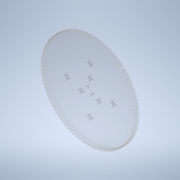
# Autodesk Inventor part: BigGear
Saved by Autodesk Inventor 2021 (Build 250183000, 183)
## iProperties
Created: 2022-02-16
Part Number: BigGear
Material: PMMA Plastic
Document SubType Name: Modeling
Designer: alexw
Mass: 170.04 g
Surface Area: 400.553 cm^2
Volume: 143.131 cm^3
Density: 1.188 g/cm^3
Appearance: Polycarbonate - Clear
BigGear_Flansch: 35,000 mm
Gear_Thick: 10,000 mm
GearDia: 162,338 mm
Dp_De_Diff_5: 1,140 mm
Author: alexw
Autodesk Inventor part; units mm, degrees
(part 1 of 2)
ref_plane "YZ Plane" through (0, 0, 0) normal (1, 0, 0) x (0, 1, 0)
ref_plane "XZ Plane" through (0, 0, 0) normal (0, 1, 0) x (-1, 0, 0)
sketch "Sketch1" plane through (0, 0, 0) normal (0, 0, 1) x (1, 0, 0)
  circle A0 centre (0, 0) radius 80.599
  circle A1 centre (0, 0) radius 6.925
  circle A2 centre (0, 0) radius 81.169 construction
  dimension "B_Gear_De" = 161.198
  dimension "d1" = 13.85
  dimension "BigGear_D" = 162.338
  constraints: 3 centre point, 3 coincident
  measures "B_Gear_De" diameter of A0
  measures "d1" diameter of A1
  measures "BigGear_D" diameter of A2
extrude "Extrusion1" add sketch "Sketch1" along normal blind 10
sketch "Sketch2" plane through (0, 0, 10) normal (0, 0, 1) x (1, 0, 0)
  line L0 (0, 17.5) -> (0, 0) construction
  circle A0 centre (0, 0) radius 17.5 construction
  point P0 (-15.1554, -8.75)
  point P1 (15.1554, -8.75)
  dimension "BigGear_Flansch" = 35
  dimension "d7" = 360
  constraints: 2 end point, 1 coincident, 1 vertical, 1 vertical alignment, 6 other
hole "Hole1" at (0, 17.5, 10) at (-15.1554, -8.75, 10) at (15.1554, -8.75, 10) direction (0, 0, -1) diameter 6.85 depth 11.8 tip angle 118
ref_plane "Work Plane1" through (0, 0, 5) normal (0, 0, 1) x (1, 0, 0)
sketch "Sketch3" plane through (0, 0, 10) normal (0, 0, 1) x (1, 0, 0)
  circle A0 centre (0, 0) radius 6.925 construction
  circle A1 centre (0, 0) radius 80.599 projected
  line L0 (0, 0) -> (0, 80.599) construction
  circle A2 centre (0, 0) radius 80.599 construction
  arc A3 (0.5699, 80.5902) -> (-0.5699, 80.5902) centre (0, 80.599) ccw construction
  arc A4 (0.5753, 80.4134) -> (2.4397, 78.6313) centre (2.4996, 80.5603) ccw
  arc A5 (-2.4397, 78.6313) -> (-0.5753, 80.4134) centre (-2.4996, 80.5603) ccw
  arc A6 (2.4996, 80.5603) -> (-2.4996, 80.5603) centre (0, 0) ccw construction
  line L1 (-2.4996, 80.5603) -> (-2.4397, 78.6313) construction
  line L2 (2.4996, 80.5603) -> (2.4397, 78.6313) construction
  line L3 (0, 80.599) -> (0, 81.169) construction
  arc A7 (2.4397, 78.6313) -> (-2.4397, 78.6313) centre (0, 0) ccw construction
  circle A8 centre (0, 0) radius 81.169 construction
  arc A9 (0.3768, 80.5981) -> (-0.3768, 80.5981) centre (0, 0) ccw
  arc A10 (-0.3768, 80.5981) -> (-0.5753, 80.4134) centre (-0.3759, 80.3981) ccw
  arc A11 (0.5753, 80.4134) -> (0.3768, 80.5981) centre (0.3759, 80.3981) ccw
  arc A12 (2.4055, 78.6323) -> (4.3761, 80.2963) centre (2.4645, 80.5613) ccw
  arc A13 (5.3378, 80.4221) -> (4.5856, 80.4685) centre (0, 0) ccw
  arc A14 (5.5245, 80.2254) -> (5.3378, 80.4221) centre (5.3245, 80.2225) ccw
  arc A15 (5.5245, 80.2254) -> (7.2757, 78.3319) centre (7.4542, 80.2536) ccw
  arc A16 (4.5856, 80.4685) -> (4.3761, 80.2963) centre (4.5742, 80.2688) ccw
  arc A17 (7.2416, 78.3351) -> (9.3109, 79.8746) centre (7.4193, 80.2568) ccw
  arc A18 (10.2785, 79.9409) -> (9.5306, 80.0336) centre (0, 0) ccw
  arc A19 (10.4528, 79.7332) -> (10.2785, 79.9409) centre (10.253, 79.7426) ccw
  arc A20 (10.4528, 79.7332) -> (12.0841, 77.7355) centre (12.3806, 79.6425) ccw
  arc A21 (9.5306, 80.0336) -> (9.3109, 79.8746) centre (9.507, 79.835) ccw
  arc A22 (12.0503, 77.7407) -> (14.2104, 79.1499) centre (12.3459, 79.6479) ccw
  arc A23 (15.1803, 79.1566) -> (14.4395, 79.295) centre (0, 0) ccw
  arc A24 (15.3414, 78.9385) -> (15.1803, 79.1566) centre (15.1426, 78.9601) ccw
  arc A25 (15.3414, 78.9385) -> (16.8467, 76.8441) centre (17.2599, 78.7293) ccw
  arc A26 (14.4395, 79.295) -> (14.2104, 79.1499) centre (14.4036, 79.0983) ccw
  arc A27 (16.8132, 76.8515) -> (19.056, 78.125) centre (17.2256, 78.7368) ccw
  arc A28 (20.0244, 78.0719) -> (19.2936, 78.2557) centre (0, 0) ccw
  arc A29 (20.1718, 77.8443) -> (20.0244, 78.0719) centre (19.9747, 77.8782) ccw
  arc A30 (20.1718, 77.8443) -> (21.5453, 75.6613) centre (22.0739, 77.5174) ccw
  arc A31 (19.2936, 78.2557) -> (19.056, 78.125) centre (19.2457, 78.0616) ccw
  arc A32 (21.5123, 75.6707) -> (23.8293, 76.8037) centre (22.0401, 77.527) ccw
  arc A33 (24.7926, 76.6911) -> (24.0745, 76.9196) centre (0, 0) ccw
  arc A34 (24.9258, 76.4549) -> (24.7926, 76.6911) centre (24.7311, 76.5008) ccw
  arc A35 (24.9258, 76.4549) -> (26.1622, 74.1914) centre (26.804, 76.0115) ccw
  arc A36 (24.0745, 76.9196) -> (23.8293, 76.8037) centre (24.0147, 76.7287) ccw
  arc A37 (26.1299, 74.2028) -> (28.5122, 75.1911) centre (26.7709, 76.0232) ccw
  arc A38 (29.4668, 75.0194) -> (28.764, 75.2916) centre (0, 0) ccw
  arc A39 (29.5851, 74.7754) -> (29.4668, 75.0194) centre (29.3937, 74.8333) ccw
  arc A40 (29.5851, 74.7754) -> (30.6799, 72.4401) centre (31.4325, 74.2172) ccw
  arc A41 (28.764, 75.2916) -> (28.5122, 75.1911) centre (28.6927, 75.1048) ccw
  arc A42 (30.6483, 72.4535) -> (33.087, 73.2932) centre (31.4002, 74.2309) ccw
  arc A43 (34.0291, 73.0631) -> (33.3445, 73.3781) centre (0, 0) ccw
  arc A44 (34.1322, 72.8123) -> (34.0291, 73.0631) centre (33.9447, 72.8818) ccw
  arc A45 (34.1322, 72.8123) -> (35.0812, 70.4141) centre (35.9418, 72.1415) ccw
  arc A46 (33.3445, 73.3781) -> (33.087, 73.2932) centre (33.2618, 73.196) ccw
  arc A47 (35.0505, 70.4293) -> (37.5362, 71.1173) centre (35.9104, 72.1571) ccw
  arc A48 (38.4624, 70.8297) -> (37.7985, 71.1862) centre (0, 0) ccw
  arc A49 (38.5499, 70.573) -> (38.4624, 70.8297) centre (38.367, 70.6539) ccw
  arc A50 (38.5499, 70.573) -> (39.3494, 68.1209) centre (40.3147, 69.792) ccw
  arc A51 (37.7985, 71.1862) -> (37.5362, 71.1173) centre (37.7047, 71.0096) ccw
  arc A52 (39.3197, 68.138) -> (41.8431, 68.6717) centre (40.2843, 69.8096) ccw
  arc A53 (42.7498, 68.3276) -> (42.1091, 68.7243) centre (0, 0) ccw
  arc A54 (42.8213, 68.066) -> (42.7498, 68.3276) centre (42.6437, 68.158) ccw
  arc A55 (42.8213, 68.066) -> (43.4684, 65.5693) centre (44.5347, 67.1778) ccw
  arc A56 (42.1091, 68.7243) -> (41.8431, 68.6717) centre (42.0046, 68.5538) ccw
  arc A57 (43.4398, 65.5882) -> (45.9912, 65.9655) centre (44.5054, 67.1972) ccw
  arc A58 (46.875, 65.5662) -> (46.2599, 66.0017) centre (0, 0) ccw
  arc A59 (46.9303, 65.3007) -> (46.875, 65.5662) centre (46.7587, 65.4035) ccw
  arc A60 (46.9303, 65.3007) -> (47.4224, 62.769) centre (48.5858, 64.3088) ccw
  arc A61 (46.2599, 66.0017) -> (45.9912, 65.9655) centre (46.1452, 65.8379) ccw
  arc A62 (47.3951, 62.7896) -> (49.9648, 63.0092) centre (48.5578, 64.33) ccw
  arc A63 (50.8225, 62.5562) -> (50.2353, 63.0287) centre (0, 0) ccw
  arc A64 (50.8613, 62.2878) -> (50.8225, 62.5562) centre (50.6963, 62.401) ccw
  arc A65 (50.8613, 62.2878) -> (51.1966, 59.7306) centre (52.4525, 61.1959) ccw
  arc A66 (50.2353, 63.0287) -> (49.9648, 63.0092) centre (50.1107, 62.8723) ccw
  arc A67 (51.1706, 59.7529) -> (53.749, 59.8138) centre (52.4259, 61.2187) ccw
  arc A68 (54.5771, 59.3089) -> (54.0201, 59.8166) centre (0, 0) ccw
  arc A69 (54.5993, 59.0386) -> (54.5771, 59.3089) centre (54.4417, 59.1617) ccw
  arc A70 (54.5993, 59.0386) -> (54.7765, 56.4656) centre (56.1203, 57.8508) ccw
  arc A71 (54.0201, 59.8166) -> (53.749, 59.8138) centre (53.8861, 59.6682) ccw
  arc A72 (54.7519, 56.4894) -> (57.3292, 56.3915) centre (56.0951, 57.8752) ccw
  arc A73 (58.1247, 55.8366) -> (57.6001, 56.3776) centre (0, 0) ccw
  arc A74 (58.1302, 55.5655) -> (58.1247, 55.8366) centre (57.9804, 55.698) ccw
  arc A75 (58.1302, 55.5655) -> (58.1487, 52.9864) centre (59.5752, 54.2862) ccw
  arc A76 (57.6001, 56.3776) -> (57.3292, 56.3915) centre (57.4571, 56.2377) ccw
  arc A77 (58.1256, 53.0117) -> (60.692, 52.7553) centre (59.5516, 54.3122) ccw
  arc A78 (61.4518, 52.1525) -> (60.9615, 52.7248) centre (0, 0) ccw
  arc A79 (61.4406, 51.8815) -> (61.4518, 52.1525) centre (61.2993, 52.0231) ccw
  arc A80 (61.4406, 51.8815) -> (61.3003, 49.3062) centre (62.8041, 50.5158) ccw
  arc A81 (60.9615, 52.7248) -> (60.692, 52.7553) centre (60.8102, 52.5939) ccw
  arc A82 (61.2788, 49.3329) -> (63.8246, 48.919) centre (62.7821, 50.5431) ccw
  arc A83 (64.5458, 48.2705) -> (64.0916, 48.8719) centre (0, 0) ccw
  arc A84 (64.5179, 48.0008) -> (64.5458, 48.2705) centre (64.3856, 48.1507) ccw
  arc A85 (64.5179, 48.0008) -> (64.2194, 45.439) centre (65.7948, 46.5537) ccw
  arc A86 (64.0916, 48.8719) -> (63.8246, 48.919) centre (63.9326, 48.7507) ccw
  arc A87 (64.1996, 45.4669) -> (66.715, 44.8971) centre (65.7745, 46.5823) ccw
  arc A88 (67.3949, 44.2055) -> (66.9787, 44.8337) centre (0, 0) ccw
  arc A89 (67.3505, 43.938) -> (67.3949, 44.2055) centre (67.2277, 44.0958) ccw
  arc A90 (67.3505, 43.938) -> (66.8949, 41.3994) centre (68.5359, 42.415) ccw
  arc A91 (66.9787, 44.8337) -> (66.715, 44.8971) centre (66.8125, 44.7225) ccw
  arc A92 (66.8768, 41.4285) -> (69.3524, 40.7049) centre (68.5174, 42.4448) ccw
  arc A93 (69.9884, 39.9727) -> (69.6116, 40.6254) centre (0, 0) ccw
  arc A94 (69.9277, 39.7085) -> (69.9884, 39.9727) centre (69.8148, 39.8736) ccw
  arc A95 (69.9277, 39.7085) -> (69.3166, 37.2028) centre (71.017, 38.1154) ccw
  arc A96 (69.6116, 40.6254) -> (69.3524, 40.7049) centre (69.4389, 40.5246) ccw
  arc A97 (69.3003, 37.233) -> (71.7267, 36.3583) centre (71.0004, 38.1463) ccw
  arc A98 (72.3165, 35.5884) -> (71.9805, 36.263) centre (0, 0) ccw
  arc A99 (72.2395, 35.3283) -> (72.3165, 35.5884) centre (72.137, 35.5001) ccw
  arc A100 (72.2395, 35.3283) -> (71.4753, 32.865) centre (73.2287, 33.6712) ccw
  arc A101 (71.9805, 36.263) -> (71.7267, 36.3583) centre (71.8019, 36.173) ccw
  arc A102 (71.461, 32.8961) -> (73.8289, 31.8738) centre (73.2141, 33.7031) ccw
  arc A103 (74.3701, 31.069) -> (74.0764, 31.763) centre (0, 0) ccw
  arc A104 (74.2774, 30.8142) -> (74.3701, 31.069) centre (74.1856, 30.9919) ccw
  arc A105 (74.2774, 30.8142) -> (73.363, 28.4026) centre (75.1627, 29.0994) ccw
  arc A106 (74.0764, 31.763) -> (73.8289, 31.8738) centre (73.8926, 31.6842) ccw
  arc A107 (73.3506, 28.4345) -> (75.651, 27.2684) centre (75.15, 29.1321) ccw
  arc A108 (76.1417, 26.4318) -> (75.8913, 27.1426) centre (0, 0) ccw
  arc A109 (76.0334, 26.1832) -> (76.1417, 26.4318) centre (75.9528, 26.3662) ccw
  arc A110 (76.0334, 26.1832) -> (74.9723, 23.8324) centre (76.8115, 24.4171) ccw
  arc A111 (75.8913, 27.1426) -> (75.651, 27.2684) centre (75.7029, 27.0752) ccw
  arc A112 (74.9619, 23.8651) -> (77.1862, 22.5595) centre (76.8009, 24.4505) ccw
  arc A113 (77.6245, 21.6943) -> (77.4182, 22.4192) centre (0, 0) ccw
  arc A114 (77.5011, 21.4528) -> (77.6245, 21.6943) centre (77.4319, 21.6405) ccw
  arc A115 (77.5011, 21.4528) -> (76.2973, 19.1719) centre (78.169, 19.6422) ccw
  arc A116 (77.4182, 22.4192) -> (77.1862, 22.5595) centre (77.2261, 22.3635) ccw
  arc A117 (76.2889, 19.2051) -> (78.4286, 17.7651) centre (78.1604, 19.6762) ccw
  arc A118 (78.8128, 16.8745) -> (78.6515, 17.6107) centre (0, 0) ccw
  arc A119 (78.6747, 16.6411) -> (78.8128, 16.8745) centre (78.6172, 16.8326) ccw
  arc A120 (78.6747, 16.6411) -> (77.3328, 14.4386) centre (79.2299, 14.7928) ccw
  arc A121 (78.6515, 17.6107) -> (78.4286, 17.7651) centre (78.4564, 17.567) ccw
  arc A122 (77.3265, 14.4723) -> (79.3735, 12.9032) centre (79.2234, 14.8273) ccw
  arc A123 (79.7021, 11.9907) -> (79.5865, 12.7354) centre (0, 0) ccw
  arc A124 (79.55, 11.7663) -> (79.7021, 11.9907) centre (79.5043, 11.961) ccw
  arc A125 (79.55, 11.7663) -> (78.075, 9.6505) centre (79.9903, 9.8873) ccw
  arc A126 (79.5865, 12.7354) -> (79.3735, 12.9032) centre (79.389, 12.7038) ccw
  arc A127 (78.0707, 9.6845) -> (80.0173, 7.9925) centre (79.986, 9.9221) ccw
  arc A128 (80.2891, 7.0615) -> (80.2196, 7.8119) centre (0, 0) ccw
  arc A129 (80.1234, 6.8468) -> (80.2891, 7.0615) centre (80.0899, 7.0439) ccw
  arc A130 (80.1234, 6.8468) -> (78.521, 4.8258) centre (80.4472, 4.9442) ccw
  arc A131 (80.2196, 7.8119) -> (80.0173, 7.9925) centre (80.0205, 7.7925) ccw
  arc A132 (78.5189, 4.86) -> (80.3575, 3.0514) centre (80.4451, 4.9793) ccw
  arc A133 (80.5715, 2.1054) -> (80.5483, 2.8587) centre (0, 0) ccw
  arc A134 (80.3929, 1.9013) -> (80.5715, 2.1054) centre (80.3716, 2.1002) ccw
  arc A135 (80.3929, 1.9013) -> (78.6691, -0.0171) centre (80.599, -0.0176) ccw
  arc A136 (80.5483, 2.8587) -> (80.3575, 3.0514) centre (80.3484, 2.8516) ccw
  arc A137 (78.6691, 0.0171) -> (80.3929, -1.9013) centre (80.599, 0.0176) ccw
  arc A138 (80.5483, -2.8587) -> (80.5715, -2.1054) centre (0, 0) ccw
  arc A139 (80.3575, -3.0514) -> (80.5483, -2.8587) centre (80.3484, -2.8516) ccw
  arc A140 (80.3575, -3.0514) -> (78.5189, -4.86) centre (80.4451, -4.9793) ccw
  arc A141 (80.5715, -2.1054) -> (80.3929, -1.9013) centre (80.3716, -2.1002) ccw
  arc A142 (78.521, -4.8258) -> (80.1234, -6.8468) centre (80.4472, -4.9442) ccw
  arc A143 (80.2196, -7.8119) -> (80.2891, -7.0615) centre (0, 0) ccw
  arc A144 (80.0173, -7.9925) -> (80.2196, -7.8119) centre (80.0205, -7.7925) ccw
  arc A145 (80.0173, -7.9925) -> (78.0707, -9.6845) centre (79.986, -9.9221) ccw
  arc A146 (80.2891, -7.0615) -> (80.1234, -6.8468) centre (80.0899, -7.0439) ccw
  arc A147 (78.075, -9.6505) -> (79.55, -11.7663) centre (79.9903, -9.8873) ccw
  arc A148 (79.5865, -12.7354) -> (79.7021, -11.9907) centre (0, 0) ccw
  arc A149 (79.3735, -12.9032) -> (79.5865, -12.7354) centre (79.389, -12.7038) ccw
  arc A150 (79.3735, -12.9032) -> (77.3265, -14.4723) centre (79.2234, -14.8273) ccw
  arc A151 (79.7021, -11.9907) -> (79.55, -11.7663) centre (79.5043, -11.961) ccw
  arc A152 (77.3328, -14.4386) -> (78.6747, -16.6411) centre (79.2299, -14.7928) ccw
  arc A153 (78.6515, -17.6107) -> (78.8128, -16.8745) centre (0, 0) ccw
  arc A154 (78.4286, -17.7651) -> (78.6515, -17.6107) centre (78.4564, -17.567) ccw
  arc A155 (78.4286, -17.7651) -> (76.2889, -19.2051) centre (78.1604, -19.6762) ccw
  arc A156 (78.8128, -16.8745) -> (78.6747, -16.6411) centre (78.6172, -16.8326) ccw
  arc A157 (76.2973, -19.1719) -> (77.5011, -21.4528) centre (78.169, -19.6422) ccw
  arc A158 (77.4182, -22.4192) -> (77.6245, -21.6943) centre (0, 0) ccw
  arc A159 (77.1862, -22.5595) -> (77.4182, -22.4192) centre (77.2261, -22.3635) ccw
  arc A160 (77.1862, -22.5595) -> (74.9619, -23.8651) centre (76.8009, -24.4505) ccw
  arc A161 (77.6245, -21.6943) -> (77.5011, -21.4528) centre (77.4319, -21.6405) ccw
  arc A162 (74.9723, -23.8324) -> (76.0334, -26.1832) centre (76.8115, -24.4171) ccw
  arc A163 (75.8913, -27.1426) -> (76.1417, -26.4318) centre (0, 0) ccw
  arc A164 (75.651, -27.2684) -> (75.8913, -27.1426) centre (75.7029, -27.0752) ccw
  arc A165 (75.651, -27.2684) -> (73.3506, -28.4345) centre (75.15, -29.1321) ccw
  arc A166 (76.1417, -26.4318) -> (76.0334, -26.1832) centre (75.9528, -26.3662) ccw
  arc A167 (73.363, -28.4026) -> (74.2774, -30.8142) centre (75.1627, -29.0994) ccw
  arc A168 (74.0764, -31.763) -> (74.3701, -31.069) centre (0, 0) ccw
  arc A169 (73.8289, -31.8738) -> (74.0764, -31.763) centre (73.8926, -31.6842) ccw
  arc A170 (73.8289, -31.8738) -> (71.461, -32.8961) centre (73.2141, -33.7031) ccw
  arc A171 (74.3701, -31.069) -> (74.2774, -30.8142) centre (74.1856, -30.9919) ccw
  arc A172 (71.4753, -32.865) -> (72.2395, -35.3283) centre (73.2287, -33.6712) ccw
  arc A173 (71.9805, -36.263) -> (72.3165, -35.5884) centre (0, 0) ccw
  arc A174 (71.7267, -36.3583) -> (71.9805, -36.263) centre (71.8019, -36.173) ccw
  arc A175 (71.7267, -36.3583) -> (69.3003, -37.233) centre (71.0004, -38.1463) ccw
  arc A176 (72.3165, -35.5884) -> (72.2395, -35.3283) centre (72.137, -35.5001) ccw
  arc A177 (69.3166, -37.2028) -> (69.9277, -39.7085) centre (71.017, -38.1154) ccw
  arc A178 (69.6116, -40.6254) -> (69.9884, -39.9727) centre (0, 0) ccw
  arc A179 (69.3524, -40.7049) -> (69.6116, -40.6254) centre (69.4389, -40.5246) ccw
  arc A180 (69.3524, -40.7049) -> (66.8768, -41.4285) centre (68.5174, -42.4448) ccw
  arc A181 (69.9884, -39.9727) -> (69.9277, -39.7085) centre (69.8148, -39.8736) ccw
  arc A182 (66.8949, -41.3994) -> (67.3505, -43.938) centre (68.5359, -42.415) ccw
  arc A183 (66.9787, -44.8337) -> (67.3949, -44.2055) centre (0, 0) ccw
  arc A184 (66.715, -44.8971) -> (66.9787, -44.8337) centre (66.8125, -44.7225) ccw
  arc A185 (66.715, -44.8971) -> (64.1996, -45.4669) centre (65.7745, -46.5823) ccw
  arc A186 (67.3949, -44.2055) -> (67.3505, -43.938) centre (67.2277, -44.0958) ccw
  arc A187 (64.2194, -45.439) -> (64.5179, -48.0008) centre (65.7948, -46.5537) ccw
  arc A188 (64.0916, -48.8719) -> (64.5458, -48.2705) centre (0, 0) ccw
  arc A189 (63.8246, -48.919) -> (64.0916, -48.8719) centre (63.9326, -48.7507) ccw
  arc A190 (63.8246, -48.919) -> (61.2788, -49.3329) centre (62.7821, -50.5431) ccw
  arc A191 (64.5458, -48.2705) -> (64.5179, -48.0008) centre (64.3856, -48.1507) ccw
  arc A192 (61.3003, -49.3062) -> (61.4406, -51.8815) centre (62.8041, -50.5158) ccw
  arc A193 (60.9615, -52.7248) -> (61.4518, -52.1525) centre (0, 0) ccw
  arc A194 (60.692, -52.7553) -> (60.9615, -52.7248) centre (60.8102, -52.5939) ccw
  arc A195 (60.692, -52.7553) -> (58.1256, -53.0117) centre (59.5516, -54.3122) ccw
  arc A196 (61.4518, -52.1525) -> (61.4406, -51.8815) centre (61.2993, -52.0231) ccw
  arc A197 (58.1487, -52.9864) -> (58.1302, -55.5655) centre (59.5752, -54.2862) ccw
  arc A198 (57.6001, -56.3776) -> (58.1247, -55.8366) centre (0, 0) ccw
  arc A199 (57.3292, -56.3915) -> (57.6001, -56.3776) centre (57.4571, -56.2377) ccw
  arc A200 (57.3292, -56.3915) -> (54.7519, -56.4894) centre (56.0951, -57.8752) ccw
  arc A201 (58.1247, -55.8366) -> (58.1302, -55.5655) centre (57.9804, -55.698) ccw
  arc A202 (54.7765, -56.4656) -> (54.5993, -59.0386) centre (56.1203, -57.8508) ccw
  arc A203 (54.0201, -59.8166) -> (54.5771, -59.3089) centre (0, 0) ccw
  arc A204 (53.749, -59.8138) -> (54.0201, -59.8166) centre (53.8861, -59.6682) ccw
  arc A205 (53.749, -59.8138) -> (51.1706, -59.7529) centre (52.4259, -61.2187) ccw
  arc A206 (54.5771, -59.3089) -> (54.5993, -59.0386) centre (54.4417, -59.1617) ccw
  arc A207 (51.1966, -59.7306) -> (50.8613, -62.2878) centre (52.4525, -61.1959) ccw
  arc A208 (50.2353, -63.0287) -> (50.8225, -62.5562) centre (0, 0) ccw
  arc A209 (49.9648, -63.0092) -> (50.2353, -63.0287) centre (50.1107, -62.8723) ccw
  arc A210 (49.9648, -63.0092) -> (47.3951, -62.7896) centre (48.5578, -64.33) ccw
  arc A211 (50.8225, -62.5562) -> (50.8613, -62.2878) centre (50.6963, -62.401) ccw
  arc A212 (47.4224, -62.769) -> (46.9303, -65.3007) centre (48.5858, -64.3088) ccw
  arc A213 (46.2599, -66.0017) -> (46.875, -65.5662) centre (0, 0) ccw
  arc A214 (45.9912, -65.9655) -> (46.2599, -66.0017) centre (46.1452, -65.8379) ccw
  arc A215 (45.9912, -65.9655) -> (43.4398, -65.5882) centre (44.5054, -67.1972) ccw
  arc A216 (46.875, -65.5662) -> (46.9303, -65.3007) centre (46.7587, -65.4035) ccw
  arc A217 (43.4684, -65.5693) -> (42.8213, -68.066) centre (44.5347, -67.1778) ccw
  arc A218 (42.1091, -68.7243) -> (42.7498, -68.3276) centre (0, 0) ccw
  arc A219 (41.8431, -68.6717) -> (42.1091, -68.7243) centre (42.0046, -68.5538) ccw
  arc A220 (41.8431, -68.6717) -> (39.3197, -68.138) centre (40.2843, -69.8096) ccw
  arc A221 (42.7498, -68.3276) -> (42.8213, -68.066) centre (42.6437, -68.158) ccw
  arc A222 (39.3494, -68.1209) -> (38.5499, -70.573) centre (40.3147, -69.792) ccw
  arc A223 (37.7985, -71.1862) -> (38.4624, -70.8297) centre (0, 0) ccw
  arc A224 (37.5362, -71.1173) -> (37.7985, -71.1862) centre (37.7047, -71.0096) ccw
  arc A225 (37.5362, -71.1173) -> (35.0505, -70.4293) centre (35.9104, -72.1571) ccw
  arc A226 (38.4624, -70.8297) -> (38.5499, -70.573) centre (38.367, -70.6539) ccw
  arc A227 (35.0812, -70.4141) -> (34.1322, -72.8123) centre (35.9418, -72.1415) ccw
  arc A228 (33.3445, -73.3781) -> (34.0291, -73.0631) centre (0, 0) ccw
  arc A229 (33.087, -73.2932) -> (33.3445, -73.3781) centre (33.2618, -73.196) ccw
  arc A230 (33.087, -73.2932) -> (30.6483, -72.4535) centre (31.4002, -74.2309) ccw
  arc A231 (34.0291, -73.0631) -> (34.1322, -72.8123) centre (33.9447, -72.8818) ccw
  arc A232 (30.6799, -72.4401) -> (29.5851, -74.7754) centre (31.4325, -74.2172) ccw
  arc A233 (28.764, -75.2916) -> (29.4668, -75.0194) centre (0, 0) ccw
  arc A234 (28.5122, -75.1911) -> (28.764, -75.2916) centre (28.6927, -75.1048) ccw
  arc A235 (28.5122, -75.1911) -> (26.1299, -74.2028) centre (26.7709, -76.0232) ccw
  arc A236 (29.4668, -75.0194) -> (29.5851, -74.7754) centre (29.3937, -74.8333) ccw
  arc A237 (26.1622, -74.1914) -> (24.9258, -76.4549) centre (26.804, -76.0115) ccw
  arc A238 (24.0745, -76.9196) -> (24.7926, -76.6911) centre (0, 0) ccw
  arc A239 (23.8293, -76.8037) -> (24.0745, -76.9196) centre (24.0147, -76.7287) ccw
  arc A240 (23.8293, -76.8037) -> (21.5123, -75.6707) centre (22.0401, -77.527) ccw
  arc A241 (24.7926, -76.6911) -> (24.9258, -76.4549) centre (24.7311, -76.5008) ccw
  arc A242 (21.5453, -75.6613) -> (20.1718, -77.8443) centre (22.0739, -77.5174) ccw
  arc A243 (19.2936, -78.2557) -> (20.0244, -78.0719) centre (0, 0) ccw
  arc A244 (19.056, -78.125) -> (19.2936, -78.2557) centre (19.2457, -78.0616) ccw
  arc A245 (19.056, -78.125) -> (16.8132, -76.8515) centre (17.2256, -78.7368) ccw
  arc A246 (20.0244, -78.0719) -> (20.1718, -77.8443) centre (19.9747, -77.8782) ccw
  arc A247 (16.8467, -76.8441) -> (15.3414, -78.9385) centre (17.2599, -78.7293) ccw
  arc A248 (14.4395, -79.295) -> (15.1803, -79.1566) centre (0, 0) ccw
  arc A249 (14.2104, -79.1499) -> (14.4395, -79.295) centre (14.4036, -79.0983) ccw
  arc A250 (14.2104, -79.1499) -> (12.0503, -77.7407) centre (12.3459, -79.6479) ccw
  arc A251 (15.1803, -79.1566) -> (15.3414, -78.9385) centre (15.1426, -78.9601) ccw
  arc A252 (12.0841, -77.7355) -> (10.4528, -79.7332) centre (12.3806, -79.6425) ccw
  arc A253 (9.5306, -80.0336) -> (10.2785, -79.9409) centre (0, 0) ccw
  arc A254 (9.3109, -79.8746) -> (9.5306, -80.0336) centre (9.507, -79.835) ccw
  arc A255 (9.3109, -79.8746) -> (7.2416, -78.3351) centre (7.4193, -80.2568) ccw
  arc A256 (10.2785, -79.9409) -> (10.4528, -79.7332) centre (10.253, -79.7426) ccw
  arc A257 (7.2757, -78.3319) -> (5.5245, -80.2254) centre (7.4542, -80.2536) ccw
  arc A258 (4.5856, -80.4685) -> (5.3378, -80.4221) centre (0, 0) ccw
  arc A259 (4.3761, -80.2963) -> (4.5856, -80.4685) centre (4.5742, -80.2688) ccw
  arc A260 (4.3761, -80.2963) -> (2.4055, -78.6323) centre (2.4645, -80.5613) ccw
  arc A261 (5.3378, -80.4221) -> (5.5245, -80.2254) centre (5.3245, -80.2225) ccw
  arc A262 (2.4397, -78.6313) -> (0.5753, -80.4134) centre (2.4996, -80.5603) ccw
  arc A263 (-0.3768, -80.5981) -> (0.3768, -80.5981) centre (0, 0) ccw
  arc A264 (-0.5753, -80.4134) -> (-0.3768, -80.5981) centre (-0.3759, -80.3981) ccw
  arc A265 (-0.5753, -80.4134) -> (-2.4397, -78.6313) centre (-2.4996, -80.5603) ccw
  arc A266 (0.3768, -80.5981) -> (0.5753, -80.4134) centre (0.3759, -80.3981) ccw
  arc A267 (-2.4055, -78.6323) -> (-4.3761, -80.2963) centre (-2.4645, -80.5613) ccw
  arc A268 (-5.3378, -80.4221) -> (-4.5856, -80.4685) centre (0, 0) ccw
  arc A269 (-5.5245, -80.2254) -> (-5.3378, -80.4221) centre (-5.3245, -80.2225) ccw
  arc A270 (-5.5245, -80.2254) -> (-7.2757, -78.3319) centre (-7.4542, -80.2536) ccw
  arc A271 (-4.5856, -80.4685) -> (-4.3761, -80.2963) centre (-4.5742, -80.2688) ccw
  arc A272 (-7.2416, -78.3351) -> (-9.3109, -79.8746) centre (-7.4193, -80.2568) ccw
  arc A273 (-10.2785, -79.9409) -> (-9.5306, -80.0336) centre (0, 0) ccw
  arc A274 (-10.4528, -79.7332) -> (-10.2785, -79.9409) centre (-10.253, -79.7426) ccw
  arc A275 (-10.4528, -79.7332) -> (-12.0841, -77.7355) centre (-12.3806, -79.6425) ccw
  arc A276 (-9.5306, -80.0336) -> (-9.3109, -79.8746) centre (-9.507, -79.835) ccw
  arc A277 (-12.0503, -77.7407) -> (-14.2104, -79.1499) centre (-12.3459, -79.6479) ccw
  arc A278 (-15.1803, -79.1566) -> (-14.4395, -79.295) centre (0, 0) ccw
  arc A279 (-15.3414, -78.9385) -> (-15.1803, -79.1566) centre (-15.1426, -78.9601) ccw
  arc A280 (-15.3414, -78.9385) -> (-16.8467, -76.8441) centre (-17.2599, -78.7293) ccw
  arc A281 (-14.4395, -79.295) -> (-14.2104, -79.1499) centre (-14.4036, -79.0983) ccw
  arc A282 (-16.8132, -76.8515) -> (-19.056, -78.125) centre (-17.2256, -78.7368) ccw
  arc A283 (-20.0244, -78.0719) -> (-19.2936, -78.2557) centre (0, 0) ccw
  arc A284 (-20.1718, -77.8443) -> (-20.0244, -78.0719) centre (-19.9747, -77.8782) ccw
  arc A285 (-20.1718, -77.8443) -> (-21.5453, -75.6613) centre (-22.0739, -77.5174) ccw
  arc A286 (-19.2936, -78.2557) -> (-19.056, -78.125) centre (-19.2457, -78.0616) ccw
  arc A287 (-21.5123, -75.6707) -> (-23.8293, -76.8037) centre (-22.0401, -77.527) ccw
  arc A288 (-24.7926, -76.6911) -> (-24.0745, -76.9196) centre (0, 0) ccw
  arc A289 (-24.9258, -76.4549) -> (-24.7926, -76.6911) centre (-24.7311, -76.5008) ccw
  arc A290 (-24.9258, -76.4549) -> (-26.1622, -74.1914) centre (-26.804, -76.0115) ccw
  arc A291 (-24.0745, -76.9196) -> (-23.8293, -76.8037) centre (-24.0147, -76.7287) ccw
  arc A292 (-26.1299, -74.2028) -> (-28.5122, -75.1911) centre (-26.7709, -76.0232) ccw
  arc A293 (-29.4668, -75.0194) -> (-28.764, -75.2916) centre (0, 0) ccw
  arc A294 (-29.5851, -74.7754) -> (-29.4668, -75.0194) centre (-29.3937, -74.8333) ccw
  arc A295 (-29.5851, -74.7754) -> (-30.6799, -72.4401) centre (-31.4325, -74.2172) ccw
  arc A296 (-28.764, -75.2916) -> (-28.5122, -75.1911) centre (-28.6927, -75.1048) ccw
  arc A297 (-30.6483, -72.4535) -> (-33.087, -73.2932) centre (-31.4002, -74.2309) ccw
  arc A298 (-34.0291, -73.0631) -> (-33.3445, -73.3781) centre (0, 0) ccw
  arc A299 (-34.1322, -72.8123) -> (-34.0291, -73.0631) centre (-33.9447, -72.8818) ccw
  arc A300 (-34.1322, -72.8123) -> (-35.0812, -70.4141) centre (-35.9418, -72.1415) ccw
  arc A301 (-33.3445, -73.3781) -> (-33.087, -73.2932) centre (-33.2618, -73.196) ccw
  arc A302 (-35.0505, -70.4293) -> (-37.5362, -71.1173) centre (-35.9104, -72.1571) ccw
  arc A303 (-38.4624, -70.8297) -> (-37.7985, -71.1862) centre (0, 0) ccw
  arc A304 (-38.5499, -70.573) -> (-38.4624, -70.8297) centre (-38.367, -70.6539) ccw
  arc A305 (-38.5499, -70.573) -> (-39.3494, -68.1209) centre (-40.3147, -69.792) ccw
  arc A306 (-37.7985, -71.1862) -> (-37.5362, -71.1173) centre (-37.7047, -71.0096) ccw
  arc A307 (-39.3197, -68.138) -> (-41.8431, -68.6717) centre (-40.2843, -69.8096) ccw
  arc A308 (-42.7498, -68.3276) -> (-42.1091, -68.7243) centre (0, 0) ccw
  arc A309 (-42.8213, -68.066) -> (-42.7498, -68.3276) centre (-42.6437, -68.158) ccw
  arc A310 (-42.8213, -68.066) -> (-43.4684, -65.5693) centre (-44.5347, -67.1778) ccw
  arc A311 (-42.1091, -68.7243) -> (-41.8431, -68.6717) centre (-42.0046, -68.5538) ccw
  arc A312 (-43.4398, -65.5882) -> (-45.9912, -65.9655) centre (-44.5054, -67.1972) ccw
  arc A313 (-46.875, -65.5662) -> (-46.2599, -66.0017) centre (0, 0) ccw
  arc A314 (-46.9303, -65.3007) -> (-46.875, -65.5662) centre (-46.7587, -65.4035) ccw
  arc A315 (-46.9303, -65.3007) -> (-47.4224, -62.769) centre (-48.5858, -64.3088) ccw
  arc A316 (-46.2599, -66.0017) -> (-45.9912, -65.9655) centre (-46.1452, -65.8379) ccw
  arc A317 (-47.3951, -62.7896) -> (-49.9648, -63.0092) centre (-48.5578, -64.33) ccw
  arc A318 (-50.8225, -62.5562) -> (-50.2353, -63.0287) centre (0, 0) ccw
  arc A319 (-50.8613, -62.2878) -> (-50.8225, -62.5562) centre (-50.6963, -62.401) ccw
  arc A320 (-50.8613, -62.2878) -> (-51.1966, -59.7306) centre (-52.4525, -61.1959) ccw
  arc A321 (-50.2353, -63.0287) -> (-49.9648, -63.0092) centre (-50.1107, -62.8723) ccw
  arc A322 (-51.1706, -59.7529) -> (-53.749, -59.8138) centre (-52.4259, -61.2187) ccw
  arc A323 (-54.5771, -59.3089) -> (-54.0201, -59.8166) centre (0, 0) ccw
  arc A324 (-54.5993, -59.0386) -> (-54.5771, -59.3089) centre (-54.4417, -59.1617) ccw
  arc A325 (-54.5993, -59.0386) -> (-54.7765, -56.4656) centre (-56.1203, -57.8508) ccw
  arc A326 (-54.0201, -59.8166) -> (-53.749, -59.8138) centre (-53.8861, -59.6682) ccw
  arc A327 (-54.7519, -56.4894) -> (-57.3292, -56.3915) centre (-56.0951, -57.8752) ccw
  arc A328 (-58.1247, -55.8366) -> (-57.6001, -56.3776) centre (0, 0) ccw
  arc A329 (-58.1302, -55.5655) -> (-58.1247, -55.8366) centre (-57.9804, -55.698) ccw
  arc A330 (-58.1302, -55.5655) -> (-58.1487, -52.9864) centre (-59.5752, -54.2862) ccw
  arc A331 (-57.6001, -56.3776) -> (-57.3292, -56.3915) centre (-57.4571, -56.2377) ccw
  arc A332 (-58.1256, -53.0117) -> (-60.692, -52.7553) centre (-59.5516, -54.3122) ccw
  arc A333 (-61.4518, -52.1525) -> (-60.9615, -52.7248) centre (0, 0) ccw
  arc A334 (-61.4406, -51.8815) -> (-61.4518, -52.1525) centre (-61.2993, -52.0231) ccw
  arc A335 (-61.4406, -51.8815) -> (-61.3003, -49.3062) centre (-62.8041, -50.5158) ccw
  arc A336 (-60.9615, -52.7248) -> (-60.692, -52.7553) centre (-60.8102, -52.5939) ccw
  arc A337 (-61.2788, -49.3329) -> (-63.8246, -48.919) centre (-62.7821, -50.5431) ccw
  arc A338 (-64.5458, -48.2705) -> (-64.0916, -48.8719) centre (0, 0) ccw
  arc A339 (-64.5179, -48.0008) -> (-64.5458, -48.2705) centre (-64.3856, -48.1507) ccw
  arc A340 (-64.5179, -48.0008) -> (-64.2194, -45.439) centre (-65.7948, -46.5537) ccw
  arc A341 (-64.0916, -48.8719) -> (-63.8246, -48.919) centre (-63.9326, -48.7507) ccw
  arc A342 (-64.1996, -45.4669) -> (-66.715, -44.8971) centre (-65.7745, -46.5823) ccw
  arc A343 (-67.3949, -44.2055) -> (-66.9787, -44.8337) centre (0, 0) ccw
  arc A344 (-67.3505, -43.938) -> (-67.3949, -44.2055) centre (-67.2277, -44.0958) ccw
  arc A345 (-67.3505, -43.938) -> (-66.8949, -41.3994) centre (-68.5359, -42.415) ccw
  arc A346 (-66.9787, -44.8337) -> (-66.715, -44.8971) centre (-66.8125, -44.7225) ccw
  arc A347 (-66.8768, -41.4285) -> (-69.3524, -40.7049) centre (-68.5174, -42.4448) ccw
  arc A348 (-69.9884, -39.9727) -> (-69.6116, -40.6254) centre (0, 0) ccw
  arc A349 (-69.9277, -39.7085) -> (-69.9884, -39.9727) centre (-69.8148, -39.8736) ccw
  arc A350 (-69.9277, -39.7085) -> (-69.3166, -37.2028) centre (-71.017, -38.1154) ccw
  arc A351 (-69.6116, -40.6254) -> (-69.3524, -40.7049) centre (-69.4389, -40.5246) ccw
  arc A352 (-69.3003, -37.233) -> (-71.7267, -36.3583) centre (-71.0004, -38.1463) ccw
  arc A353 (-72.3165, -35.5884) -> (-71.9805, -36.263) centre (0, 0) ccw
  arc A354 (-72.2395, -35.3283) -> (-72.3165, -35.5884) centre (-72.137, -35.5001) ccw
  arc A355 (-72.2395, -35.3283) -> (-71.4753, -32.865) centre (-73.2287, -33.6712) ccw
  arc A356 (-71.9805, -36.263) -> (-71.7267, -36.3583) centre (-71.8019, -36.173) ccw
  arc A357 (-71.461, -32.8961) -> (-73.8289, -31.8738) centre (-73.2141, -33.7031) ccw
  arc A358 (-74.3701, -31.069) -> (-74.0764, -31.763) centre (0, 0) ccw
  arc A359 (-74.2774, -30.8142) -> (-74.3701, -31.069) centre (-74.1856, -30.9919) ccw
  arc A360 (-74.2774, -30.8142) -> (-73.363, -28.4026) centre (-75.1627, -29.0994) ccw
  arc A361 (-74.0764, -31.763) -> (-73.8289, -31.8738) centre (-73.8926, -31.6842) ccw
  arc A362 (-73.3506, -28.4345) -> (-75.651, -27.2684) centre (-75.15, -29.1321) ccw
  arc A363 (-76.1417, -26.4318) -> (-75.8913, -27.1426) centre (0, 0) ccw
  arc A364 (-76.0334, -26.1832) -> (-76.1417, -26.4318) centre (-75.9528, -26.3662) ccw
  arc A365 (-76.0334, -26.1832) -> (-74.9723, -23.8324) centre (-76.8115, -24.4171) ccw
  arc A366 (-75.8913, -27.1426) -> (-75.651, -27.2684) centre (-75.7029, -27.0752) ccw
  arc A367 (-74.9619, -23.8651) -> (-77.1862, -22.5595) centre (-76.8009, -24.4505) ccw
  arc A368 (-77.6245, -21.6943) -> (-77.4182, -22.4192) centre (0, 0) ccw
  arc A369 (-77.5011, -21.4528) -> (-77.6245, -21.6943) centre (-77.4319, -21.6405) ccw
  arc A370 (-77.5011, -21.4528) -> (-76.2973, -19.1719) centre (-78.169, -19.6422) ccw
  arc A371 (-77.4182, -22.4192) -> (-77.1862, -22.5595) centre (-77.2261, -22.3635) ccw
  arc A372 (-76.2889, -19.2051) -> (-78.4286, -17.7651) centre (-78.1604, -19.6762) ccw
  arc A373 (-78.8128, -16.8745) -> (-78.6515, -17.6107) centre (0, 0) ccw
  arc A374 (-78.6747, -16.6411) -> (-78.8128, -16.8745) centre (-78.6172, -16.8326) ccw
  arc A375 (-78.6747, -16.6411) -> (-77.3328, -14.4386) centre (-79.2299, -14.7928) ccw
  arc A376 (-78.6515, -17.6107) -> (-78.4286, -17.7651) centre (-78.4564, -17.567) ccw
  arc A377 (-77.3265, -14.4723) -> (-79.3735, -12.9032) centre (-79.2234, -14.8273) ccw
  arc A378 (-79.7021, -11.9907) -> (-79.5865, -12.7354) centre (0, 0) ccw
  arc A379 (-79.55, -11.7663) -> (-79.7021, -11.9907) centre (-79.5043, -11.961) ccw
  arc A380 (-79.55, -11.7663) -> (-78.075, -9.6505) centre (-79.9903, -9.8873) ccw
  arc A381 (-79.5865, -12.7354) -> (-79.3735, -12.9032) centre (-79.389, -12.7038) ccw
  arc A382 (-78.0707, -9.6845) -> (-80.0173, -7.9925) centre (-79.986, -9.9221) ccw
  arc A383 (-80.2891, -7.0615) -> (-80.2196, -7.8119) centre (0, 0) ccw
  arc A384 (-80.1234, -6.8468) -> (-80.2891, -7.0615) centre (-80.0899, -7.0439) ccw
  arc A385 (-80.1234, -6.8468) -> (-78.521, -4.8258) centre (-80.4472, -4.9442) ccw
  arc A386 (-80.2196, -7.8119) -> (-80.0173, -7.9925) centre (-80.0205, -7.7925) ccw
  arc A387 (-78.5189, -4.86) -> (-80.3575, -3.0514) centre (-80.4451, -4.9793) ccw
  arc A388 (-80.5715, -2.1054) -> (-80.5483, -2.8587) centre (0, 0) ccw
  arc A389 (-80.3929, -1.9013) -> (-80.5715, -2.1054) centre (-80.3716, -2.1002) ccw
  arc A390 (-80.3929, -1.9013) -> (-78.6691, 0.0171) centre (-80.599, 0.0176) ccw
  arc A391 (-80.5483, -2.8587) -> (-80.3575, -3.0514) centre (-80.3484, -2.8516) ccw
  arc A392 (-78.6691, -0.0171) -> (-80.3929, 1.9013) centre (-80.599, -0.0176) ccw
  arc A393 (-80.5483, 2.8587) -> (-80.5715, 2.1054) centre (0, 0) ccw
  arc A394 (-80.3575, 3.0514) -> (-80.5483, 2.8587) centre (-80.3484, 2.8516) ccw
  arc A395 (-80.3575, 3.0514) -> (-78.5189, 4.86) centre (-80.4451, 4.9793) ccw
  arc A396 (-80.5715, 2.1054) -> (-80.3929, 1.9013) centre (-80.3716, 2.1002) ccw
  arc A397 (-78.521, 4.8258) -> (-80.1234, 6.8468) centre (-80.4472, 4.9442) ccw
  arc A398 (-80.2196, 7.8119) -> (-80.2891, 7.0615) centre (0, 0) ccw
  arc A399 (-80.0173, 7.9925) -> (-80.2196, 7.8119) centre (-80.0205, 7.7925) ccw
  arc A400 (-80.0173, 7.9925) -> (-78.0707, 9.6845) centre (-79.986, 9.9221) ccw
  arc A401 (-80.2891, 7.0615) -> (-80.1234, 6.8468) centre (-80.0899, 7.0439) ccw
  arc A402 (-78.075, 9.6505) -> (-79.55, 11.7663) centre (-79.9903, 9.8873) ccw
  arc A403 (-79.5865, 12.7354) -> (-79.7021, 11.9907) centre (0, 0) ccw
  arc A404 (-79.3735, 12.9032) -> (-79.5865, 12.7354) centre (-79.389, 12.7038) ccw
  arc A405 (-79.3735, 12.9032) -> (-77.3265, 14.4723) centre (-79.2234, 14.8273) ccw
  arc A406 (-79.7021, 11.9907) -> (-79.55, 11.7663) centre (-79.5043, 11.961) ccw
  arc A407 (-77.3328, 14.4386) -> (-78.6747, 16.6411) centre (-79.2299, 14.7928) ccw
  arc A408 (-78.6515, 17.6107) -> (-78.8128, 16.8745) centre (0, 0) ccw
  arc A409 (-78.4286, 17.7651) -> (-78.6515, 17.6107) centre (-78.4564, 17.567) ccw
  arc A410 (-78.4286, 17.7651) -> (-76.2889, 19.2051) centre (-78.1604, 19.6762) ccw
  arc A411 (-78.8128, 16.8745) -> (-78.6747, 16.6411) centre (-78.6172, 16.8326) ccw
  arc A412 (-76.2973, 19.1719) -> (-77.5011, 21.4528) centre (-78.169, 19.6422) ccw
  arc A413 (-77.4182, 22.4192) -> (-77.6245, 21.6943) centre (0, 0) ccw
  arc A414 (-77.1862, 22.5595) -> (-77.4182, 22.4192) centre (-77.2261, 22.3635) ccw
  arc A415 (-77.1862, 22.5595) -> (-74.9619, 23.8651) centre (-76.8009, 24.4505) ccw
  arc A416 (-77.6245, 21.6943) -> (-77.5011, 21.4528) centre (-77.4319, 21.6405) ccw
  arc A417 (-74.9723, 23.8324) -> (-76.0334, 26.1832) centre (-76.8115, 24.4171) ccw
  arc A418 (-75.8913, 27.1426) -> (-76.1417, 26.4318) centre (0, 0) ccw
  arc A419 (-75.651, 27.2684) -> (-75.8913, 27.1426) centre (-75.7029, 27.0752) ccw
  arc A420 (-75.651, 27.2684) -> (-73.3506, 28.4345) centre (-75.15, 29.1321) ccw
  arc A421 (-76.1417, 26.4318) -> (-76.0334, 26.1832) centre (-75.9528, 26.3662) ccw
  arc A422 (-73.363, 28.4026) -> (-74.2774, 30.8142) centre (-75.1627, 29.0994) ccw
  arc A423 (-74.0764, 31.763) -> (-74.3701, 31.069) centre (0, 0) ccw
  arc A424 (-73.8289, 31.8738) -> (-74.0764, 31.763) centre (-73.8926, 31.6842) ccw
  arc A425 (-73.8289, 31.8738) -> (-71.461, 32.8961) centre (-73.2141, 33.7031) ccw
  arc A426 (-74.3701, 31.069) -> (-74.2774, 30.8142) centre (-74.1856, 30.9919) ccw
  arc A427 (-71.4753, 32.865) -> (-72.2395, 35.3283) centre (-73.2287, 33.6712) ccw
  arc A428 (-71.9805, 36.263) -> (-72.3165, 35.5884) centre (0, 0) ccw
  arc A429 (-71.7267, 36.3583) -> (-71.9805, 36.263) centre (-71.8019, 36.173) ccw
  arc A430 (-71.7267, 36.3583) -> (-69.3003, 37.233) centre (-71.0004, 38.1463) ccw
  arc A431 (-72.3165, 35.5884) -> (-72.2395, 35.3283) centre (-72.137, 35.5001) ccw
  arc A432 (-69.3166, 37.2028) -> (-69.9277, 39.7085) centre (-71.017, 38.1154) ccw
  arc A433 (-69.6116, 40.6254) -> (-69.9884, 39.9727) centre (0, 0) ccw
  arc A434 (-69.3524, 40.7049) -> (-69.6116, 40.6254) centre (-69.4389, 40.5246) ccw
  arc A435 (-69.3524, 40.7049) -> (-66.8768, 41.4285) centre (-68.5174, 42.4448) ccw
  arc A436 (-69.9884, 39.9727) -> (-69.9277, 39.7085) centre (-69.8148, 39.8736) ccw
  arc A437 (-66.8949, 41.3994) -> (-67.3505, 43.938) centre (-68.5359, 42.415) ccw
  arc A438 (-66.9787, 44.8337) -> (-67.3949, 44.2055) centre (0, 0) ccw
  arc A439 (-66.715, 44.8971) -> (-66.9787, 44.8337) centre (-66.8125, 44.7225) ccw
  arc A440 (-66.715, 44.8971) -> (-64.1996, 45.4669) centre (-65.7745, 46.5823) ccw
  arc A441 (-67.3949, 44.2055) -> (-67.3505, 43.938) centre (-67.2277, 44.0958) ccw
  arc A442 (-64.2194, 45.439) -> (-64.5179, 48.0008) centre (-65.7948, 46.5537) ccw
  arc A443 (-64.0916, 48.8719) -> (-64.5458, 48.2705) centre (0, 0) ccw
  arc A444 (-63.8246, 48.919) -> (-64.0916, 48.8719) centre (-63.9326, 48.7507) ccw
  arc A445 (-63.8246, 48.919) -> (-61.2788, 49.3329) centre (-62.7821, 50.5431) ccw
  arc A446 (-64.5458, 48.2705) -> (-64.5179, 48.0008) centre (-64.3856, 48.1507) ccw
  arc A447 (-61.3003, 49.3062) -> (-61.4406, 51.8815) centre (-62.8041, 50.5158) ccw
  arc A448 (-60.9615, 52.7248) -> (-61.4518, 52.1525) centre (0, 0) ccw
  arc A449 (-60.692, 52.7553) -> (-60.9615, 52.7248) centre (-60.8102, 52.5939) ccw
  arc A450 (-60.692, 52.7553) -> (-58.1256, 53.0117) centre (-59.5516, 54.3122) ccw
  arc A451 (-61.4518, 52.1525) -> (-61.4406, 51.8815) centre (-61.2993, 52.0231) ccw
  arc A452 (-58.1487, 52.9864) -> (-58.1302, 55.5655) centre (-59.5752, 54.2862) ccw
  arc A453 (-57.6001, 56.3776) -> (-58.1247, 55.8366) centre (0, 0) ccw
  arc A454 (-57.3292, 56.3915) -> (-57.6001, 56.3776) centre (-57.4571, 56.2377) ccw
  arc A455 (-57.3292, 56.3915) -> (-54.7519, 56.4894) centre (-56.0951, 57.8752) ccw
  arc A456 (-58.1247, 55.8366) -> (-58.1302, 55.5655) centre (-57.9804, 55.698) ccw
  arc A457 (-54.7765, 56.4656) -> (-54.5993, 59.0386) centre (-56.1203, 57.8508) ccw
  arc A458 (-54.0201, 59.8166) -> (-54.5771, 59.3089) centre (0, 0) ccw
  arc A459 (-53.749, 59.8138) -> (-54.0201, 59.8166) centre (-53.8861, 59.6682) ccw
  arc A460 (-53.749, 59.8138) -> (-51.1706, 59.7529) centre (-52.4259, 61.2187) ccw
  arc A461 (-54.5771, 59.3089) -> (-54.5993, 59.0386) centre (-54.4417, 59.1617) ccw
  arc A462 (-51.1966, 59.7306) -> (-50.8613, 62.2878) centre (-52.4525, 61.1959) ccw
  arc A463 (-50.2353, 63.0287) -> (-50.8225, 62.5562) centre (0, 0) ccw
  arc A464 (-49.9648, 63.0092) -> (-50.2353, 63.0287) centre (-50.1107, 62.8723) ccw
  arc A465 (-49.9648, 63.0092) -> (-47.3951, 62.7896) centre (-48.5578, 64.33) ccw
  arc A466 (-50.8225, 62.5562) -> (-50.8613, 62.2878) centre (-50.6963, 62.401) ccw
  arc A467 (-47.4224, 62.769) -> (-46.9303, 65.3007) centre (-48.5858, 64.3088) ccw
  arc A468 (-46.2599, 66.0017) -> (-46.875, 65.5662) centre (0, 0) ccw
  arc A469 (-45.9912, 65.9655) -> (-46.2599, 66.0017) centre (-46.1452, 65.8379) ccw
  arc A470 (-45.9912, 65.9655) -> (-43.4398, 65.5882) centre (-44.5054, 67.1972) ccw
  arc A471 (-46.875, 65.5662) -> (-46.9303, 65.3007) centre (-46.7587, 65.4035) ccw
  arc A472 (-43.4684, 65.5693) -> (-42.8213, 68.066) centre (-44.5347, 67.1778) ccw
  arc A473 (-42.1091, 68.7243) -> (-42.7498, 68.3276) centre (0, 0) ccw
  arc A474 (-41.8431, 68.6717) -> (-42.1091, 68.7243) centre (-42.0046, 68.5538) ccw
  arc A475 (-41.8431, 68.6717) -> (-39.3197, 68.138) centre (-40.2843, 69.8096) ccw
  arc A476 (-42.7498, 68.3276) -> (-42.8213, 68.066) centre (-42.6437, 68.158) ccw
  arc A477 (-39.3494, 68.1209) -> (-38.5499, 70.573) centre (-40.3147, 69.792) ccw
  arc A478 (-37.7985, 71.1862) -> (-38.4624, 70.8297) centre (0, 0) ccw
  arc A479 (-37.5362, 71.1173) -> (-37.7985, 71.1862) centre (-37.7047, 71.0096) ccw
  arc A480 (-37.5362, 71.1173) -> (-35.0505, 70.4293) centre (-35.9104, 72.1571) ccw
  arc A481 (-38.4624, 70.8297) -> (-38.5499, 70.573) centre (-38.367, 70.6539) ccw
  arc A482 (-35.0812, 70.4141) -> (-34.1322, 72.8123) centre (-35.9418, 72.1415) ccw
  arc A483 (-33.3445, 73.3781) -> (-34.0291, 73.0631) centre (0, 0) ccw
  arc A484 (-33.087, 73.2932) -> (-33.3445, 73.3781) centre (-33.2618, 73.196) ccw
  arc A485 (-33.087, 73.2932) -> (-30.6483, 72.4535) centre (-31.4002, 74.2309) ccw
  arc A486 (-34.0291, 73.0631) -> (-34.1322, 72.8123) centre (-33.9447, 72.8818) ccw
  arc A487 (-30.6799, 72.4401) -> (-29.5851, 74.7754) centre (-31.4325, 74.2172) ccw
  arc A488 (-28.764, 75.2916) -> (-29.4668, 75.0194) centre (0, 0) ccw
  arc A489 (-28.5122, 75.1911) -> (-28.764, 75.2916) centre (-28.6927, 75.1048) ccw
  arc A490 (-28.5122, 75.1911) -> (-26.1299, 74.2028) centre (-26.7709, 76.0232) ccw
  arc A491 (-29.4668, 75.0194) -> (-29.5851, 74.7754) centre (-29.3937, 74.8333) ccw
  arc A492 (-26.1622, 74.1914) -> (-24.9258, 76.4549) centre (-26.804, 76.0115) ccw
  arc A493 (-24.0745, 76.9196) -> (-24.7926, 76.6911) centre (0, 0) ccw
  arc A494 (-23.8293, 76.8037) -> (-24.0745, 76.9196) centre (-24.0147, 76.7287) ccw
  arc A495 (-23.8293, 76.8037) -> (-21.5123, 75.6707) centre (-22.0401, 77.527) ccw
  arc A496 (-24.7926, 76.6911) -> (-24.9258, 76.4549) centre (-24.7311, 76.5008) ccw
  arc A497 (-21.5453, 75.6613) -> (-20.1718, 77.8443) centre (-22.0739, 77.5174) ccw
  arc A498 (-19.2936, 78.2557) -> (-20.0244, 78.0719) centre (0, 0) ccw
  arc A499 (-19.056, 78.125) -> (-19.2936, 78.2557) centre (-19.2457, 78.0616) ccw
  arc A500 (-19.056, 78.125) -> (-16.8132, 76.8515) centre (-17.2256, 78.7368) ccw
  arc A501 (-20.0244, 78.0719) -> (-20.1718, 77.8443) centre (-19.9747, 77.8782) ccw
  arc A502 (-16.8467, 76.8441) -> (-15.3414, 78.9385) centre (-17.2599, 78.7293) ccw
  arc A503 (-14.4395, 79.295) -> (-15.1803, 79.1566) centre (0, 0) ccw
  arc A504 (-14.2104, 79.1499) -> (-14.4395, 79.295) centre (-14.4036, 79.0983) ccw
  arc A505 (-14.2104, 79.1499) -> (-12.0503, 77.7407) centre (-12.3459, 79.6479) ccw
  arc A506 (-15.1803, 79.1566) -> (-15.3414, 78.9385) centre (-15.1426, 78.9601) ccw
  arc A507 (-12.0841, 77.7355) -> (-10.4528, 79.7332) centre (-12.3806, 79.6425) ccw
  arc A508 (-9.5306, 80.0336) -> (-10.2785, 79.9409) centre (0, 0) ccw
  arc A509 (-9.3109, 79.8746) -> (-9.5306, 80.0336) centre (-9.507, 79.835) ccw
  arc A510 (-9.3109, 79.8746) -> (-7.2416, 78.3351) centre (-7.4193, 80.2568) ccw
  arc A511 (-10.2785, 79.9409) -> (-10.4528, 79.7332) centre (-10.253, 79.7426) ccw
  arc A512 (-7.2757, 78.3319) -> (-5.5245, 80.2254) centre (-7.4542, 80.2536) ccw
  arc A513 (-4.5856, 80.4685) -> (-5.3378, 80.4221) centre (0, 0) ccw
  arc A514 (-4.3761, 80.2963) -> (-4.5856, 80.4685) centre (-4.5742, 80.2688) ccw
  arc A515 (-4.3761, 80.2963) -> (-2.4055, 78.6323) centre (-2.4645, 80.5613) ccw
  arc A516 (-5.3378, 80.4221) -> (-5.5245, 80.2254) centre (-5.3245, 80.2225) ccw
  point P0 (0, 78.6691)
  point P1 (4.3924, 80.4724)
  point P2 (4.9617, 80.4462)
  point P3 (5.5301, 80.4022)
  point P4 (9.338, 80.0494)
  point P5 (9.9047, 79.9881)
  point P6 (10.4692, 79.9093)
  point P7 (14.2482, 79.3227)
  point P8 (14.81, 79.2267)
  point P9 (15.3686, 79.1133)
  point P10 (19.1043, 78.2951)
  point P11 (19.6592, 78.1647)
  point P12 (20.2098, 78.0171)
  point P13 (23.888, 76.9705)
  point P14 (24.4338, 76.8062)
  point P15 (24.9742, 76.625)
  point P16 (28.5811, 75.354)
  point P17 (29.1157, 75.1563)
  point P18 (29.644, 74.9422)
  point P19 (33.1657, 73.4516)
  point P20 (33.6872, 73.2214)
  point P21 (34.2013, 72.9752)
  point P22 (37.6246, 71.2706)
  point P23 (38.1309, 71.0087)
  point P24 (38.6288, 70.7313)
  point P25 (41.9407, 68.8192)
  point P26 (42.4299, 68.5267)
  point P27 (42.9098, 68.2191)
  point P28 (46.0977, 66.1067)
  point P29 (46.568, 65.7847)
  point P30 (47.0281, 65.4482)
  point P31 (50.0799, 63.1435)
  point P32 (50.5294, 62.7931)
  point P33 (50.9679, 62.4289)
  point P34 (53.8721, 59.9408)
  point P35 (54.2992, 59.5634)
  point P36 (54.7144, 59.1729)
  point P37 (57.4599, 56.5107)
  point P38 (57.863, 56.1077)
  point P39 (58.2534, 55.6924)
  point P40 (60.8298, 52.8663)
  point P41 (61.2073, 52.4392)
  point P42 (61.5714, 52.0006)
  point P43 (63.9689, 49.0212)
  point P44 (64.3194, 48.5718)
  point P45 (64.6558, 48.1116)
  point P46 (66.8654, 44.9903)
  point P47 (67.1875, 44.5201)
  point P48 (67.495, 44.0401)
  point P49 (69.5082, 40.7887)
  point P50 (69.8008, 40.2995)
  point P51 (70.0781, 39.8015)
  point P52 (71.8873, 36.4323)
  point P53 (72.1493, 35.9261)
  point P54 (72.3954, 35.412)
  point P55 (73.9938, 31.9378)
  point P56 (74.2241, 31.4164)
  point P57 (74.4381, 30.8881)
  point P58 (75.8196, 27.3221)
  point P59 (76.0173, 26.7875)
  point P60 (76.1984, 26.247)
  point P61 (77.3577, 22.6027)
  point P62 (77.5222, 22.057)
  point P63 (77.6697, 21.5064)
  point P64 (78.6025, 17.7976)
  point P65 (78.733, 17.2428)
  point P66 (78.8463, 16.6842)
  point P67 (79.549, 12.925)
  point P68 (79.6452, 12.3632)
  point P69 (79.7239, 11.7987)
  point P70 (80.1938, 8.0034)
  point P71 (80.2552, 7.4367)
  point P72 (80.299, 6.8684)
  point P73 (80.5344, 3.0514)
  point P74 (80.5608, 2.4821)
  point P75 (80.5695, 1.9121)
  point P76 (80.5695, -1.9121)
  point P77 (80.5608, -2.4821)
  point P78 (80.5344, -3.0514)
  point P79 (80.299, -6.8684)
  point P80 (80.2552, -7.4367)
  point P81 (80.1938, -8.0034)
  point P82 (79.7239, -11.7987)
  point P83 (79.6452, -12.3632)
  point P84 (79.549, -12.925)
  point P85 (78.8463, -16.6842)
  point P86 (78.733, -17.2428)
  point P87 (78.6025, -17.7976)
  point P88 (77.6697, -21.5064)
  point P89 (77.5222, -22.057)
  point P90 (77.3577, -22.6027)
  point P91 (76.1984, -26.247)
  point P92 (76.0173, -26.7875)
  point P93 (75.8196, -27.3221)
  point P94 (74.4381, -30.8881)
  point P95 (74.2241, -31.4164)
  point P96 (73.9938, -31.9378)
  point P97 (72.3954, -35.412)
  point P98 (72.1493, -35.9261)
  point P99 (71.8873, -36.4323)
  point P100 (70.0781, -39.8015)
  point P101 (69.8008, -40.2995)
  point P102 (69.5082, -40.7887)
  point P103 (67.495, -44.0401)
  point P104 (67.1875, -44.5201)
  point P105 (66.8654, -44.9903)
  point P106 (64.6558, -48.1116)
  point P107 (64.3194, -48.5718)
  point P108 (63.9689, -49.0212)
  point P109 (61.5714, -52.0006)
  point P110 (61.2073, -52.4392)
  point P111 (60.8298, -52.8663)
  point P112 (58.2534, -55.6924)
  point P113 (57.863, -56.1077)
  point P114 (57.4599, -56.5107)
  point P115 (54.7144, -59.1729)
  point P116 (54.2992, -59.5634)
  point P117 (53.8721, -59.9408)
  point P118 (50.9679, -62.4289)
  point P119 (50.5294, -62.7931)
  point P120 (50.0799, -63.1435)
  point P121 (47.0281, -65.4482)
  point P122 (46.568, -65.7847)
  point P123 (46.0977, -66.1067)
  point P124 (42.9098, -68.2191)
  point P125 (42.4299, -68.5267)
  point P126 (41.9407, -68.8192)
  point P127 (38.6288, -70.7313)
  point P128 (38.1309, -71.0087)
  point P129 (37.6246, -71.2706)
  point P130 (34.2013, -72.9752)
  point P131 (33.6872, -73.2214)
  point P132 (33.1657, -73.4516)
  point P133 (29.644, -74.9422)
  point P134 (29.1157, -75.1563)
  point P135 (28.5811, -75.354)
  point P136 (24.9742, -76.625)
  point P137 (24.4338, -76.8062)
  point P138 (23.888, -76.9705)
  point P139 (20.2098, -78.0171)
  point P140 (19.6592, -78.1647)
  point P141 (19.1043, -78.2951)
  point P142 (15.3686, -79.1133)
  point P143 (14.81, -79.2267)
  point P144 (14.2482, -79.3227)
  point P145 (10.4692, -79.9093)
  point P146 (9.9047, -79.9881)
  point P147 (9.338, -80.0494)
  point P148 (5.5301, -80.4022)
  point P149 (4.9617, -80.4462)
  point P150 (4.3924, -80.4724)
  point P151 (0.5699, -80.5902)
  point P152 (0, -80.599)
  point P153 (-0.5699, -80.5902)
  point P154 (-4.3924, -80.4724)
  point P155 (-4.9617, -80.4462)
  point P156 (-5.5301, -80.4022)
  point P157 (-9.338, -80.0494)
  point P158 (-9.9047, -79.9881)
  point P159 (-10.4692, -79.9093)
  point P160 (-14.2482, -79.3227)
  point P161 (-14.81, -79.2267)
  point P162 (-15.3686, -79.1133)
  point P163 (-19.1043, -78.2951)
  point P164 (-19.6592, -78.1647)
  point P165 (-20.2098, -78.0171)
  point P166 (-23.888, -76.9705)
  point P167 (-24.4338, -76.8062)
  point P168 (-24.9742, -76.625)
  point P169 (-28.5811, -75.354)
  point P170 (-29.1157, -75.1563)
  point P171 (-29.644, -74.9422)
  point P172 (-33.1657, -73.4516)
  point P173 (-33.6872, -73.2214)
  point P174 (-34.2013, -72.9752)
  point P175 (-37.6246, -71.2706)
  point P176 (-38.1309, -71.0087)
  point P177 (-38.6288, -70.7313)
  point P178 (-41.9407, -68.8192)
  point P179 (-42.4299, -68.5267)
  point P180 (-42.9098, -68.2191)
  point P181 (-46.0977, -66.1067)
  point P182 (-46.568, -65.7847)
  point P183 (-47.0281, -65.4482)
  point P184 (-50.0799, -63.1435)
  point P185 (-50.5294, -62.7931)
  point P186 (-50.9679, -62.4289)
  point P187 (-53.8721, -59.9408)
  point P188 (-54.2992, -59.5634)
  point P189 (-54.7144, -59.1729)